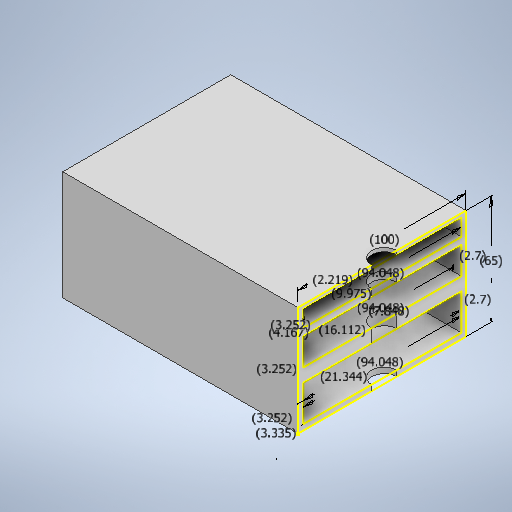
# Autodesk Inventor part: hddcase
Saved by Autodesk Inventor 2025.1 (Build 291241000, 241)
## iProperties
Created: 2024-10-03
Part Number: hddcase
Material: Generic
Document SubType Name: Modeling
Designer: tidal
Density: 1 g/cm^3
Appearance: Default
Author: tidal
Autodesk Inventor part; units mm, degrees
ref_plane "YZ Plane" through (0, 0, 0) normal (1, 0, 0) x (0, 1, 0)
ref_plane "XZ Plane" through (0, 0, 0) normal (0, 1, 0) x (-1, 0, 0)
ref_plane "XY Plane" through (0, 0, 0) normal (0, 0, 1) x (1, 0, 0)
sketch "Sketch1" plane through (0, 0, 0) normal (0, 1, 0) x (-1, 0, 0)
  point P0 (0, 0)
sketch "Sketch2" plane through (0, 0, 0) normal (0, 1, 0) x (-1, 0, 0)
  point P0 (0, 0)
sketch "Sketch3" plane through (0, 0, 0) normal (0, 1, 0) x (-1, 0, 0)
  line L0 (0, 0) -> (140, 0)
  line L1 (140, 0) -> (140, -100)
  line L2 (140, -100) -> (0, -100)
  line L3 (0, -100) -> (0, 0)
  dimension "d0" = 140
  dimension "d1" = 100
  constraints: 8 end point, 2 parallel, 1 horizontal, 1 perpendicular
  measures "d0" distance of L1.end L2.end
  measures "d1" distance of L0.end L1.end
extrude "Extrusion1" add sketch "Sketch3" along normal blind 65
sketch "Sketch4" plane through (0, 0, 0) normal (1, 0, 0) x (0, 0, -1)
  line L0 (3.2517, 3.335) -> (97.2996, 3.335)
  line L1 (97.2996, 3.335) -> (97.2996, 24.6792)
  line L2 (97.2996, 24.6792) -> (3.2517, 24.6792)
  line L3 (3.2517, 24.6792) -> (3.2517, 3.335)
  point P0 (0, 0)
  constraints: 8 end point, 2 parallel, 1 horizontal, 1 perpendicular
extrude "Extrusion2" cut sketch "Sketch4" against normal blind 136.85
sketch "Sketch6" plane through (0, 0, 0) normal (1, 0, 0) x (0, 0, -1)
  line L0 (3.2517, 32.5271) -> (97.2996, 32.5271)
  line L1 (97.2996, 32.5271) -> (97.2996, 48.6393)
  line L2 (97.2996, 48.6393) -> (3.2517, 48.6393)
  line L3 (3.2517, 48.6393) -> (3.2517, 32.5271)
  point P0 (0, 0)
  constraints: 8 end point, 2 parallel, 1 horizontal, 1 perpendicular
extrude "Extrusion4" cut sketch "Sketch6" against normal blind 135.4125
sketch "Sketch7" plane through (0, 0, 0) normal (1, 0, 0) x (0, 0, -1)
  line L0 (3.2517, 52.8064) -> (97.2996, 52.8064)
  line L1 (97.2996, 52.8064) -> (97.2996, 62.7809)
  line L2 (97.2996, 62.7809) -> (3.2517, 62.7809)
  line L3 (3.2517, 62.7809) -> (3.2517, 52.8064)
  point P0 (0, 0)
  constraints: 8 end point, 2 parallel, 1 horizontal, 1 perpendicular
extrude "Extrusion5" cut sketch "Sketch7" against normal blind 134.85
sketch "Sketch8" plane through (0, 0, 0) normal (1, 0, 0) x (0, 0, -1)
  line L0 (97.2996, 62.7809) -> (97.2996, 52.8064) projected
  line L1 (3.2517, 52.8064) -> (3.2517, 62.7809) projected
  line L2 (97.2996, 52.8064) -> (3.2517, 52.8064) projected
  line L3 (3.2517, 62.7809) -> (97.2996, 62.7809) projected
  line L4 (97.2996, 32.5271) -> (3.2517, 32.5271) projected
  line L5 (3.2517, 48.6393) -> (97.2996, 48.6393) projected
  line L6 (97.2996, 48.6393) -> (97.2996, 32.5271) projected
  line L7 (3.2517, 32.5271) -> (3.2517, 48.6393) projected
  line L8 (97.2996, 24.6792) -> (97.2996, 3.335) projected
  line L9 (3.2517, 3.335) -> (3.2517, 24.6792) projected
  line L10 (97.2996, 3.335) -> (3.2517, 3.335) projected
  line L11 (3.2517, 24.6792) -> (97.2996, 24.6792) projected
  point P0 (0, 0)
  point P1 (3.2517, 57.7937)
  dimension "d20" = 94.048
  dimension "d21" = 9.9745
  dimension "d22" = 16.1122
  dimension "d23" = 94.048
  dimension "d24" = 94.048
  dimension "d25" = 21.3442
  constraints: 1 midpoint
  measures "d20" distance from line of L0 point (3.252, 57.794)
  measures "d21" distance between parallel lines of L2 L3
  measures "d22" distance between parallel lines of L4 L5
  measures "d23" distance between parallel lines of L6 L7
  measures "d24" distance between parallel lines of L8 L9
  measures "d25" distance between parallel lines of L10 L11
sketch "Sketch9" plane through (0, 0, 0) normal (1, 0, 0) x (0, 0, -1)
  line L0 (100, 0) -> (100, 65) projected
  line L1 (0, 0) -> (0, 65) projected
  line L2 (0, 0) -> (100, 0) projected
  line L3 (0, 65) -> (100, 65) projected
  line L4 (3.2517, 62.7809) -> (97.2996, 62.7809) projected
  line L5 (3.2517, 52.8064) -> (3.2517, 62.7809) projected
  line L6 (3.2517, 48.6393) -> (97.2996, 48.6393) projected
  line L7 (97.2996, 52.8064) -> (3.2517, 52.8064) projected
  line L8 (3.2517, 32.5271) -> (3.2517, 48.6393) projected
  line L9 (3.2517, 24.6792) -> (97.2996, 24.6792) projected
  line L10 (97.2996, 32.5271) -> (3.2517, 32.5271) projected
  line L11 (97.2996, 48.6393) -> (97.2996, 32.5271) projected
  line L12 (3.2517, 3.335) -> (3.2517, 24.6792) projected
  line L13 (97.2996, 24.6792) -> (97.2996, 3.335) projected
  line L14 (97.2996, 3.335) -> (3.2517, 3.335) projected
  dimension "d26" = 100
  dimension "d27" = 65
  dimension "d28" = 2.2191
  dimension "d29" = 3.2517
  dimension "d30" = 4.167
  dimension "d31" = 3.2517
  dimension "d32" = 7.8479
  dimension "d33" = 2.7004
  dimension "d34" = 3.2517
  dimension "d35" = 2.7004
  dimension "d36" = 3.335
  measures "d26" distance between parallel lines of L0 L1
  measures "d27" distance between parallel lines of L2 L3
  measures "d28" distance between parallel lines of L4 L3
  measures "d29" distance between parallel lines of L5 L1
  measures "d30" distance between parallel lines of L6 L7
  measures "d31" distance between parallel lines of L1 L8
  measures "d32" distance between parallel lines of L9 L10
  measures "d33" distance between parallel lines of L0 L11
  measures "d34" distance between parallel lines of L1 L12
  measures "d35" distance between parallel lines of L0 L13
  measures "d36" distance between parallel lines of L14 L2
sketch "Sketch10" plane through (0, 65, 0) normal (0, 1, 0) x (1, 0, 0)
  line L0 (0, 0) -> (0, 100) projected
  circle A0 centre (0, 51.3457) radius 7.5
  point P0 (0, 58.8457)
  point P1 (0, 43.8457)
  dimension "d37" = 15
  constraints: 1 centre point, 1 point on line
  measures "d37" diameter of A0
extrude "Extrusion6" cut sketch "Sketch10" against normal blind 65 contours A0 L0 picked at (-3.0801, 51.117)
body "Solid1"
